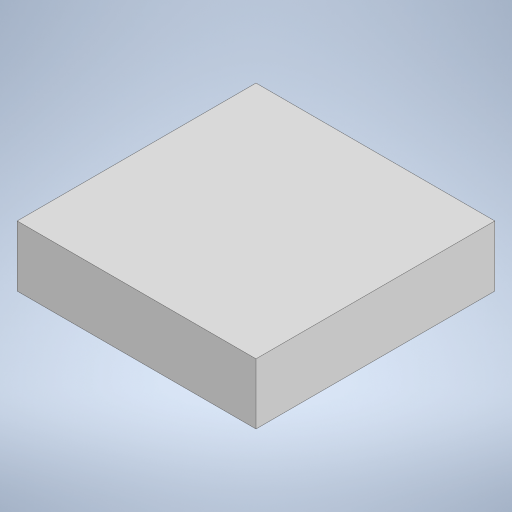
# Autodesk Inventor part: silicon_mold
Saved by Autodesk Inventor 2023.1 (Build 271208000, 208)
## iProperties
Created: 2022-08-08
Part Number: silicon_mold
Material: Generic
Document SubType Name: Modeling
Designer: fraaw
Density: 1 g/cm^3
Appearance: Default
Author: fraaw
## iProperties of the stored document silicon_mold_3DPrint.ipt
Created: 2022-08-08
Part Number: silicon_mold_3DPrint
Material: Generic
Document SubType Name: Modeling
Designer: fraaw
Density: 1 g/cm^3
Appearance: Default
Author: fraaw
Autodesk Inventor part; units mm, degrees
ref_plane "YZ Plane" through (0, 0, 0) normal (1, 0, 0) x (0, 1, 0)
ref_plane "XZ Plane" through (0, 0, 0) normal (0, 1, 0) x (-1, 0, 0)
ref_plane "XY Plane" through (0, 0, 0) normal (0, 0, 1) x (1, 0, 0)
sketch "Sketch1" plane through (0, 0, 0) normal (0, 1, 0) x (-1, 0, 0)
  line L0 (-14.75, 14.75) -> (14.75, 14.75)
  line L1 (14.75, 14.75) -> (14.75, -14.75)
  line L2 (14.75, -14.75) -> (-14.75, -14.75)
  line L3 (-14.75, -14.75) -> (-14.75, 14.75)
  line L4 (-14.75, 14.75) -> (14.75, -14.75) construction
  line L5 (14.75, 14.75) -> (-14.75, -14.75) construction
  line L6 (13.75, 13.75) -> (-13.75, 13.75)
  line L7 (-13.75, 13.75) -> (-13.75, -13.75)
  line L8 (-13.75, -13.75) -> (13.75, -13.75)
  line L9 (13.75, -13.75) -> (13.75, 13.75)
  point P0 (0, 0)
  dimension "d0" = 29.5
  dimension "d1" = 29.5
  dimension "d2" = 1
  constraints: 20 end point, 4 parallel, 2 midpoint, 2 perpendicular, 1 horizontal, 3 other
  measures "d0" distance of L0.end L1.end
  measures "d1" distance of L0.start L0.end
  measures "d2" distance between parallel lines of L0 L6
extrude "Extrusion1" add sketch "Sketch1" along normal blind 5.5
sketch "Sketch2" plane through (0, 5.5, 0) normal (0, 1, 0) x (1, 0, 0)
  line L0 (-14.75, 14.75) -> (-14.75, -14.75) projected
  line L1 (-14.75, -14.75) -> (14.75, -14.75) projected
  line L2 (14.75, -14.75) -> (14.75, 14.75) projected
  line L3 (14.75, 14.75) -> (-14.75, 14.75) projected
  point P0 (0, 0)
extrude "Extrusion2" add sketch "Sketch2" along normal blind 2
sketch "Sketch3" plane through (0, 5.5, 0) normal (0, -1, 0) x (1, 0, 0)
  line L0 (-13.75, 13.75) -> (-13.75, -13.75) projected
  line L1 (13.75, 13.75) -> (-13.75, 13.75) projected
  point P0 (0, 0)
  point P1 (-11, 11)
  point P2 (-8.25, 11)
  point P3 (-5.5, 11)
  point P4 (-2.75, 11)
  point P5 (0, 11)
  point P6 (2.75, 11)
  point P7 (5.5, 11)
  point P8 (8.25, 11)
  point P9 (11, 11)
  point P10 (-11, 8.25)
  point P11 (-8.25, 8.25)
  point P12 (-5.5, 8.25)
  point P13 (-2.75, 8.25)
  point P14 (0, 8.25)
  point P15 (2.75, 8.25)
  point P16 (5.5, 8.25)
  point P17 (8.25, 8.25)
  point P18 (11, 8.25)
  point P19 (-11, 5.5)
  point P20 (-8.25, 5.5)
  point P21 (-5.5, 5.5)
  point P22 (-2.75, 5.5)
  point P23 (0, 5.5)
  point P24 (2.75, 5.5)
  point P25 (5.5, 5.5)
  point P26 (8.25, 5.5)
  point P27 (11, 5.5)
  point P28 (-11, 2.75)
  point P29 (-8.25, 2.75)
  point P30 (-5.5, 2.75)
  point P31 (-2.75, 2.75)
  point P32 (0, 2.75)
  point P33 (2.75, 2.75)
  point P34 (5.5, 2.75)
  point P35 (8.25, 2.75)
  point P36 (11, 2.75)
  point P37 (-11, 0)
  point P38 (-8.25, 0)
  point P39 (-5.5, 0)
  point P40 (-2.75, 0)
  point P41 (0, 0)
  point P42 (2.75, 0)
  point P43 (5.5, 0)
  point P44 (8.25, 0)
  point P45 (11, 0)
  point P46 (-11, -2.75)
  point P47 (-8.25, -2.75)
  point P48 (-5.5, -2.75)
  point P49 (-2.75, -2.75)
  point P50 (0, -2.75)
  point P51 (2.75, -2.75)
  point P52 (5.5, -2.75)
  point P53 (8.25, -2.75)
  point P54 (11, -2.75)
  point P55 (-11, -5.5)
  point P56 (-8.25, -5.5)
  point P57 (-5.5, -5.5)
  point P58 (-2.75, -5.5)
  point P59 (0, -5.5)
  point P60 (2.75, -5.5)
  point P61 (5.5, -5.5)
  point P62 (8.25, -5.5)
  point P63 (11, -5.5)
  point P64 (-11, -8.25)
  point P65 (-8.25, -8.25)
  point P66 (-5.5, -8.25)
  point P67 (-2.75, -8.25)
  point P68 (0, -8.25)
  point P69 (2.75, -8.25)
  point P70 (5.5, -8.25)
  point P71 (8.25, -8.25)
  point P72 (11, -8.25)
  point P73 (-11, -11)
  point P74 (-8.25, -11)
  point P75 (-5.5, -11)
  point P76 (-2.75, -11)
  point P77 (0, -11)
  point P78 (2.75, -11)
  point P79 (5.5, -11)
  point P80 (8.25, -11)
  point P81 (11, -11)
  dimension "d7" = 2.75
  dimension "d8" = 2.75
  dimension "d11" = 2.75
  dimension "d14" = 2.75
  constraints: 1 horizontal, 1 vertical, 80 other
  measures "d7" distance from line of L0 point (-11, 11)
  measures "d8" distance from line of L1 point (-11, 11)
  measures "d11" distance of point (-11, 11) point (-8.25, 11)
  measures "d14" distance of point (-11, 11) point (-11, 8.25)
hole "Hole1" at (-11, 5.5, 11) at (-8.25, 5.5, 11) at (-5.5, 5.5, 11) at (-2.75, 5.5, 11) at (0, 5.5, 11) at (2.75, 5.5, 11) at (5.5, 5.5, 11) at (8.25, 5.5, 11) at (11, 5.5, 11) at (-11, 5.5, 8.25) at (-8.25, 5.5, 8.25) at (-5.5, 5.5, 8.25) at (-2.75, 5.5, 8.25) at (0, 5.5, 8.25) at (2.75, 5.5, 8.25) at (5.5, 5.5, 8.25) at (8.25, 5.5, 8.25) at (11, 5.5, 8.25) at (-11, 5.5, 5.5) at (-8.25, 5.5, 5.5) at (-5.5, 5.5, 5.5) at (-2.75, 5.5, 5.5) at (0, 5.5, 5.5) at (2.75, 5.5, 5.5) at (5.5, 5.5, 5.5) at (8.25, 5.5, 5.5) at (11, 5.5, 5.5) at (-11, 5.5, 2.75) at (-8.25, 5.5, 2.75) at (-5.5, 5.5, 2.75) at (-2.75, 5.5, 2.75) at (0, 5.5, 2.75) at (2.75, 5.5, 2.75) at (5.5, 5.5, 2.75) at (8.25, 5.5, 2.75) at (11, 5.5, 2.75) at (-11, 5.5, 0) at (-8.25, 5.5, 0) at (-5.5, 5.5, 0) at (-2.75, 5.5, 0) at (0, 5.5, 0) at (2.75, 5.5, 0) at (5.5, 5.5, 0) at (8.25, 5.5, 0) at (11, 5.5, 0) at (-11, 5.5, -2.75) at (-8.25, 5.5, -2.75) at (-5.5, 5.5, -2.75) at (-2.75, 5.5, -2.75) at (0, 5.5, -2.75) direction (0, 1, 0) diameter 1.5 depth 0.5 and at (2.75, 5.5, -2.75) (5.5, 5.5, -2.75) (8.25, 5.5, -2.75) (11, 5.5, -2.75) (-11, 5.5, -5.5) (-8.25, 5.5, -5.5) (-5.5, 5.5, -5.5) (-2.75, 5.5, -5.5) (0, 5.5, -5.5) (2.75, 5.5, -5.5) (5.5, 5.5, -5.5) (8.25, 5.5, -5.5) (11, 5.5, -5.5) (-11, 5.5, -8.25) (-8.25, 5.5, -8.25) (-5.5, 5.5, -8.25) (-2.75, 5.5, -8.25) (0, 5.5, -8.25) (2.75, 5.5, -8.25) (5.5, 5.5, -8.25) (8.25, 5.5, -8.25) (11, 5.5, -8.25) (-11, 5.5, -11) (-8.25, 5.5, -11) (-5.5, 5.5, -11) (-2.75, 5.5, -11) (0, 5.5, -11) (2.75, 5.5, -11) (5.5, 5.5, -11) (8.25, 5.5, -11) (11, 5.5, -11)
fillet "Fillet1" radius 0.5 1 edges at (-11, 6, 11.75)
pattern_linear "Rectangular Pattern1" count 9 spacing 2.75 along (1, 0, 0) count 9 spacing 2.75 along (0, 0, -1) of "Fillet1"
equation "\"d1\" = d0"
body "Solid1"
